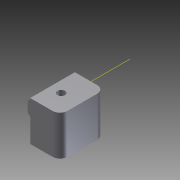
# Autodesk Inventor part: bolt mount
Saved by Autodesk Inventor 2012 (Build 160160000, 160)
## iProperties
Created: 2012-01-05
Part Number: bolt mount
Material: Default
Document SubType Name: Modeling
Designer: Kennell
Density: 1 g/cm^3
Author: Kennell
Autodesk Inventor part; units mm, degrees
ref_plane "YZ Plane" through (0, 0, 0) normal (1, 0, 0) x (0, 1, 0)
ref_plane "XZ Plane" through (0, 0, 0) normal (0, 1, 0) x (-1, 0, 0)
ref_plane "XY Plane" through (0, 0, 0) normal (0, 0, 1) x (1, 0, 0)
sketch "Sketch1" plane through (0, 0, 0) normal (0, 0, 1) x (1, 0, 0)
  line L0 (0, 0) -> (21.5, 0)
  line L1 (21.5, 0) -> (21.5, 18)
  line L2 (21.5, 18) -> (9.5, 18)
  line L3 (9.5, 18) -> (9.5, 9.5)
  line L4 (9.5, 9.5) -> (0, 9.5)
  line L5 (0, 9.5) -> (0, 0)
  dimension "d0" = 9.5
  dimension "d1" = 9.5
  dimension "d2" = 18
  dimension "d3" = 12
  constraints: 12 end point, 3 parallel, 2 perpendicular, 1 horizontal
  measures "d0" distance of L4.end L0.start
  measures "d1" distance of L3.end L4.end
  measures "d2" distance of L0.end L1.end
  measures "d3" distance of L1.end L2.end
extrude "Extrusion1" add sketch "Sketch1" along normal blind 8
sketch "Sketch2" plane through (0, 0, 8) normal (0, 0, 1) x (1, 0, 0)
  line L0 (21.5, 0) -> (0, 0) projected
  line L1 (9.5, 9.5) -> (9.5, 18) projected
  line L2 (21.5, 18) -> (9.5, 18)
  line L3 (9.5, 18) -> (9.5, 0)
  line L4 (9.5, 0) -> (21.5, 0)
  line L5 (21.5, 0) -> (21.5, 18)
  constraints: 8 end point, 2 parallel, 1 collinear, 1 horizontal, 1 perpendicular, 1 point on line
extrude "Extrusion2" add sketch "Sketch2" along normal blind 8
hole "Hole1" at (4, 0, 4) direction (0, 1, 0) diameter 3 end through all
chamfer "Chamfer1" distance 2 angle 45 2 edges at (0, 4.75, 8) (0, 4.75, 0)
fillet "Fillet1" radius 3 2 edges at (21.5, 0, 8) (21.5, 18, 8)
hole "Hole2" at (14, 10, 16) direction (0, 0, -1) diameter 3 end through all
ref_plane "Work Plane1" through (9.5, -5, 8) normal (0, -1, 0) x (1, 0, 0)
mirror "Mirror1" about plane through (9.5, -5, 8) normal (0, -1, 0) remove original yes
hole "Hole4" at (14, -20, 0) direction (0, 0, 1) diameter 6 depth 2
body "Solid1"
